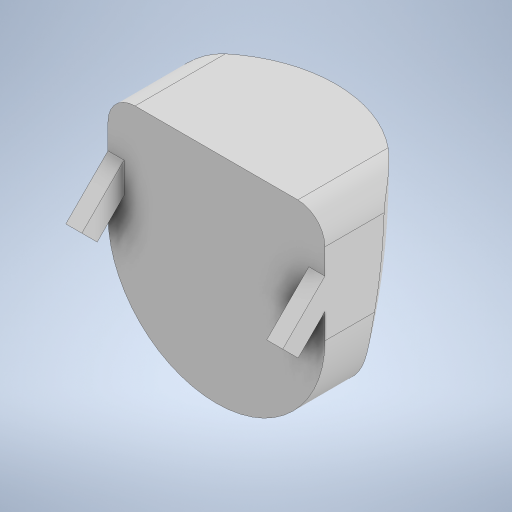
# Autodesk Inventor part: FingerTip Hardtip
Saved by Autodesk Inventor 2023 (Build 270158000, 158)
## iProperties
Created: 2023-04-11
Part Number: FingerTip Hardtip
Material: Generic
Document SubType Name: Modeling
Designer: 1roweste
Density: 1 g/cm^3
Appearance: Default
Author: 1roweste
Autodesk Inventor part; units mm, degrees
ref_plane "YZ Plane" through (0, 0, 0) normal (1, 0, 0) x (0, 1, 0)
sketch "Imprint Transfer" plane through (0, 0, 0) normal (0, 0, 1) x (1, 0, 0)
  arc A0 (-10, 10) -> (10, 10) centre (0, 10) ccw
  line L0 (10, 10) -> (10, 17.5)
  arc A1 (10, 17.5) -> (7.5, 20) centre (7.5, 17.5) ccw
  line L1 (7.5, 20) -> (-7.5, 20)
  arc A2 (-7.5, 20) -> (-10, 17.5) centre (-7.5, 17.5) ccw
  line L2 (-10, 17.5) -> (-10, 10)
  point P0 (0, 0)
  point P1 (0, 7.0711)
  constraints: 6 end point, 6 point on circle, 3 centre point
sketch "Sketch2" plane through (0, 0, 0) normal (0, 0, 1) x (1, 0, 0)
  line L0 (-10, 17.5) -> (-10, 10) projected
  arc A0 (-10, 10) -> (10, 10) centre (0, 10) ccw projected
  line L1 (10, 10) -> (10, 17.5) projected
  arc A1 (10, 17.5) -> (7.5, 20) centre (7.5, 17.5) ccw projected
  line L2 (7.5, 20) -> (-7.5, 20) projected
  arc A2 (-7.5, 20) -> (-10, 17.5) centre (-7.5, 17.5) ccw projected
  point P0 (0, 0)
extrude "Extrusion1" add sketch "Sketch2" against normal blind 11
sketch "Rotational Axis" plane through (0, 0, 0) normal (0, 0, 1) x (1, 0, 0)
  arc A0 (-10, 10) -> (10, 10) centre (0, 10) ccw projected
  line L0 (10, 10) -> (10, 17.5) projected
  arc A1 (10, 17.5) -> (7.5, 20) centre (7.5, 17.5) ccw projected
  line L1 (7.5, 20) -> (-7.5, 20) projected
  arc A2 (-7.5, 20) -> (-10, 17.5) centre (-7.5, 17.5) ccw projected
  line L2 (-10, 17.5) -> (-10, 10) projected
  line L3 (-10, 10) -> (-10, 17.5) projected
  line L4 (-10, 13.75) -> (10, 13.75)
  line L5 (10, 17.5) -> (10, 10) projected
  point P0 (0, 0)
  constraints: 2 end point, 2 midpoint
ref_plane "Dovetail Plane" through (-10, 13.75, 0) normal (0, -0.7071068, 0.7071068) x (1, 0, 0)
sketch "Sketch4" plane through (-10, 13.75, 0) normal (0, -0.7071068, 0.7071068) x (1, 0, 0)
  ellipse E0 centre (10, -2.6517) end of major axis (0, -2.6517) minor radius 7.0711 (0, -2.6517) -> (20, -2.6517) ccw projected
  line L0 (20, -2.6517) -> (20, 2.6517) projected
  ellipse E1 centre (17.5, 2.6517) end of major axis (20, 2.6517) minor radius 1.7678 (20, 2.6517) -> (17.5, 4.4194) ccw projected
  line L1 (17.5, 4.4194) -> (2.5, 4.4194) projected
  ellipse E2 centre (2.5, 2.6517) end of major axis (0, 2.6517) minor radius 1.7678 (2.5, 4.4194) -> (0, 2.6517) ccw projected
  line L2 (0, 2.6517) -> (0, -2.6517) projected
  line L3 (0, 0) -> (20, 0)
  line L4 (0, 1) -> (20, 1)
  line L5 (0, -1) -> (20, -1)
  line L6 (0, 1) -> (1.48, 1)
  line L7 (1.48, 1) -> (1.48, -1)
  line L8 (1.48, -1) -> (0, -1)
  line L9 (0, -1) -> (0, 1)
  line L10 (20, 1) -> (18.52, 1)
  line L11 (18.52, 1) -> (18.52, -1)
  line L12 (18.52, -1) -> (20, -1)
  line L13 (20, -1) -> (20, 1)
  point P0 (10, -9.7227)
  point P1 (1.48, 1)
  point P2 (0, 1)
  point P3 (0, -1)
  point P4 (1.48, -1)
  point P5 (18.52, 1)
  point P6 (18.52, -1)
  point P7 (20, -1)
  point P8 (20, 1)
  dimension "d3" = 1
  dimension "d4" = 1
  dimension "d5" = 1.48
  dimension "d6" = 2
  dimension "d7" = 1.48
  dimension "d8" = 2
  dimension "d13" = 0
  dimension "d14" = 0
  constraints: 22 end point, 6 parallel, 2 horizontal, 2 midpoint, 2 perpendicular, 3 other
  measures "d3" distance between parallel lines of L3 L4
  measures "d4" distance between parallel lines of L3 L5
  measures "d5" distance of L7.end L8.end
  measures "d6" distance of L6.end L7.end
  measures "d7" distance of L12.end L11.end
  measures "d8" distance of L11.end L10.end
  measures "d13" distance between parallel lines of L0 L13
  measures "d14" distance between parallel lines of L2 L9
extrude "Extrusion2" add sketch "Sketch4" along normal blind 4.5 and the other way blind 2 contours L2 L3 L7 L5 | L5 L11 L3 L0 | L2 L4 L7 L3 | L3 L11 L4 L0
sketch "Sketch6" plane through (-7.5, 20, 0) normal (0, 1, 0) x (1, 0, 0)
  line L0 (15, 0) -> (0, 0) projected
  line L1 (15, 0) -> (15, 11) projected
  line L2 (0, 11) -> (15, 11) projected
  line L3 (0, 0) -> (0, 11) projected
  line L4 (17.5, 0) -> (15, 0) projected
  line L5 (17.5, 0) -> (17.5, 11) projected
  line L6 (15, 11) -> (17.5, 11) projected
  line L7 (15, 0) -> (15, 11) projected
  line L8 (0, 0) -> (-2.5, 0) projected
  line L9 (0, 0) -> (0, 11) projected
  line L10 (-2.5, 11) -> (0, 11) projected
  line L11 (-2.5, 0) -> (-2.5, 11) projected
  line L12 (17.5, 0) -> (17.5, 11) projected
  line L13 (-2.5, 0) -> (-2.5, 11) projected
  arc A0 (17.5, 5.5) -> (-2.5, 5.5) centre (7.5, -0.8409) ccw
  line L14 (17.5, 11) -> (-2.5, 11)
  line L15 (-2.5, 11) -> (-2.5, 16)
  line L16 (-2.5, 16) -> (17.5, 16)
  line L17 (17.5, 16) -> (17.5, 11)
  point P0 (7.5, 0)
  point P1 (7.5, 11)
  point P2 (-2.5, 5.5)
  dimension "d27" = 20
  dimension "d28" = 5
  constraints: 8 end point, 2 midpoint, 2 parallel, 2 point on circle, 1 centre point, 1 horizontal, 1 perpendicular
  measures "d27" distance of L15.end L16.end
  measures "d28" distance of L14.end L15.end
ref_plane "MidPlane" through (0, 10, -11) normal (1, 0, 0) x (0, 0, -1)
sketch "GuideReference" plane through (0, 10, -11) normal (1, 0, 0) x (0, 0, -1)
  line L0 (-11, 0) -> (-11, 0) projected
  line L1 (-11, 0) -> (0, 0) projected
  line L2 (0, 0) -> (0, 0) projected
  line L3 (-11, 0) -> (0, 0) projected
  line L4 (-11, 10) -> (-11, 7.5) projected
  line L5 (-11, 10) -> (0, 10) projected
  line L6 (0, 7.5) -> (0, 10) projected
  line L7 (-11, 7.5) -> (0, 7.5) projected
  line L8 (-11, 7.5) -> (-11, 5.1642) projected
  line L9 (-11, 7.5) -> (0, 7.5) projected
  line L10 (0, 0) -> (0, 7.5) projected
  line L11 (-11, 0) -> (0, 0) projected
  line L12 (-11, 2.3358) -> (-11, 0) projected
  line L13 (-11, 2.3358) -> (-13.4749, -0.1391) projected
  line L14 (-14.8891, 1.2751) -> (-13.4749, -0.1391) projected
  line L15 (-11, 5.1642) -> (-14.8891, 1.2751) projected
  line L16 (-11.8409, -10) -> (-0.8409, -10) construction
  line L17 (-11.8409, 10) -> (-11.8409, -7.5)
  line L18 (-11.8409, 10) -> (5.6591, 10) construction
  line L19 (-11.8409, -7.5) -> (-18.8409, -7.5)
  line L20 (-18.8409, -7.5) -> (-22.8409, -7.5)
  line L21 (-11.8409, 10) -> (-11.8409, -7.5) construction
  line L22 (-11.8409, -7.5) -> (-18.8409, -7.5) construction
  line L23 (-18.8409, -7.5) -> (-22.8409, -7.5) construction
  spline S0 degree 3 poles (-11.8409, 10) (-11.8409, -7.5) (-18.8409, -7.5) (-22.8409, -7.5) knots 1 1 1 1 2 2 2 2
  point P0 (-11, -10)
  dimension "d24" = 17.5
  dimension "d25" = 90
  dimension "d26" = 7
  constraints: 10 end point, 3 perpendicular, 2 coincident, 2 collinear, 2 horizontal, 1 point on line, 3 other
  measures "d24" distance of L17.start L17.end
  measures "d25" angle of L17 L18
  measures "d26" distance of L17.end L19.end
sketch "Sketch10" plane through (0, 10, -11) normal (1, 0, 0) x (0, 0, -1)
  spline S0 degree 3 poles (-11.8409, 10) (-11.8409, -7.5) (-18.8409, -7.5) (-22.8409, -7.5) knots 1 1 1 1 2 2 2 2 projected
  point P0 (-11, -10)
sweep "Sweep2" cut profiles "Sketch6" path "Sketch10" contours A0 L2 L1 | L1 L6 L5 A0 | A0 L11 L10 L3 | L3 L2 A0 | L2 L10 L15 L16 L17 L6
body "Solid1"
